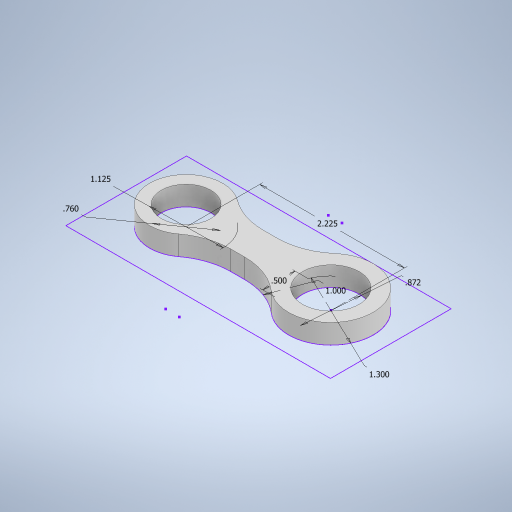
# Autodesk Inventor part: C.Connecting Rod Cutting Jig
Saved by Autodesk Inventor 2023 (Build 270158000, 158)
## iProperties
Created: 2022-10-29
Part Number: C.Connecting Rod Cutting Jig
Material: Generic
Document SubType Name: Modeling
Designer: tommy
Density: 1 g/cm^3
Appearance: Default
Author: tommy
Autodesk Inventor part; units mm, degrees
ref_plane "YZ Plane" through (0, 0, 0) normal (1, 0, 0) x (0, 1, 0)
ref_plane "XZ Plane" through (0, 0, 0) normal (0, 1, 0) x (-1, 0, 0)
ref_plane "XY Plane" through (0, 0, 0) normal (0, 0, 1) x (1, 0, 0)
sketch "Sketch1" plane through (0, 0, 0) normal (0, 1, 0) x (-1, 0, 0)
  circle A0 centre (-31.75, 0) radius 11.0744
  circle A1 centre (24.765, 0) radius 9.652
  line L0 (-4.3934, -6.35) -> (0.9525, -6.35)
  arc A2 (16.1925, -11.43) -> (16.1925, 11.43) centre (24.765, 0) ccw
  arc A3 (-20.9731, 12.5076) -> (-20.9731, -12.5076) centre (-31.75, 0) ccw
  line L1 (-4.3934, 6.35) -> (0.9525, 6.35)
  line L2 (-54.5659, 23.0342) -> (48.7426, 23.0342)
  line L3 (48.7426, 23.0342) -> (48.7426, -24.079)
  line L4 (48.7426, -24.079) -> (-54.5659, -24.079)
  line L5 (-54.5659, -24.079) -> (-54.5659, 23.0342)
  arc A4 (-20.9731, 12.5076) -> (-4.3934, 6.35) centre (-4.3934, 31.75) ccw
  arc A5 (0.9525, 6.35) -> (16.1925, 11.43) centre (0.9525, 31.75) ccw
  arc A6 (16.1925, -11.43) -> (0.9525, -6.35) centre (0.9525, -31.75) ccw
  arc A7 (-4.3934, -6.35) -> (-20.9731, -12.5076) centre (-4.3934, -31.75) ccw
  point P0 (0, 0)
  point P1 (-16.51, -6.35)
  point P2 (-16.51, 6.35)
  point P3 (11.9662, -6.35)
  point P4 (11.9662, 6.35)
  dimension "d15" = 22.1488
  dimension "d17" = 12.7
  dimension "d18" = 33.02
  dimension "d19" = 19.304
  dimension "d20" = 28.575
  dimension "d21" = 56.515
  dimension "d35" = 25.4
  constraints: 16 point on circle, 12 end point, 8 centre point, 8 tangent, 4 point on line, 3 equal radius, 2 horizontal, 2 parallel, 1 coincident, 1 concentric, 1 perpendicular
  measures "d15" diameter of A0
  measures "d17" distance of point (-16.51, -6.35) point (-16.51, 6.35)
  measures "d18" diameter of A3
  measures "d19" diameter of A1
  measures "d20" diameter of A2
  measures "d21" distance of A1.centre A0.centre
  measures "d35" radius of A4
extrude "Extrusion2" add sketch "Sketch1" along normal blind 7.62 contours A7 A3 A4 L1 A5 A2 A6 L0
body "Solid2"
